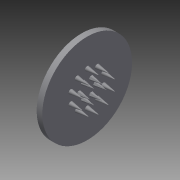
# Autodesk Inventor part: foam gripper
Saved by Autodesk Inventor 2015 (Build 190159000, 159)
## iProperties
Created: 2014-11-02
Part Number: foam gripper
Material: Generic
Document SubType Name: Modeling
Designer: jesse
Density: 1 g/cm^3
Appearance: Default
Author: jesse
Autodesk Inventor part; units mm, degrees
ref_plane "YZ Plane" through (0, 0, 0) normal (1, 0, 0) x (0, 1, 0)
ref_plane "XZ Plane" through (0, 0, 0) normal (0, 1, 0) x (-1, 0, 0)
ref_plane "XY Plane" through (0, 0, 0) normal (0, 0, 1) x (1, 0, 0)
sketch "Sketch1" plane through (0, 0, 0) normal (1, 0, 0) x (0, 1, 0)
  circle A0 centre (0, 0) radius 50.8
  dimension "d0" = 101.6
  constraints: 1 centre point, 1 coincident
  measures "d0" diameter of A0
extrude "Extrusion1" add sketch "Sketch1" along normal blind 3.175
sketch "Sketch2" plane through (3.175, 0, 0) normal (1, 0, 0) x (0, 0, -1)
  circle A0 centre (0, 19.4049) radius 2.54
  point P0 (0, 0)
  dimension "d3" = 5.08
  constraints: 1 centre point
  measures "d3" diameter of A0
extrude "Extrusion2" add sketch "Sketch2" along normal blind 12.7 draft -10
pattern_circular "Circular Pattern1" count 10 over 360 about axis through (0, 0, 0) along (1, 0, 0) of "Extrusion2"
sketch "Sketch3" plane through (3.175, 0, 0) normal (1, 0, 0) x (0, 0, -1)
  line L0 (6.7407, 0) -> (8.0059, 2.1913)
  line L1 (8.0059, 2.1913) -> (10.5361, 2.1913)
  line L2 (10.5361, 2.1913) -> (11.8012, 0)
  line L3 (11.8012, 0) -> (10.5361, -2.1913)
  line L4 (10.5361, -2.1913) -> (8.0059, -2.1913)
  line L5 (8.0059, -2.1913) -> (6.7407, 0)
  point P0 (0, 0)
  point P1 (9.271, 0)
  constraints: 12 end point, 13 other
extrude "Extrusion3" add sketch "Sketch3" along normal blind 12.7 draft -10
pattern_circular "Circular Pattern2" count 6 over 360 about axis through (0, 0, 0) along (1, 0, 0) of "Extrusion3"
sketch "Sketch4" plane through (3.175, 0, 0) normal (1, 0, 0) x (0, 0, -1)
  line L0 (-5.461, 3.1529) -> (0, 6.3058)
  line L1 (0, 6.3058) -> (5.461, 3.1529)
  line L2 (5.461, 3.1529) -> (5.461, -3.1529)
  line L3 (5.461, -3.1529) -> (0, -6.3058)
  line L4 (0, -6.3058) -> (-5.461, -3.1529)
  line L5 (-5.461, -3.1529) -> (-5.461, 3.1529)
  line L6 (-7.0782, -4.0866) -> (0, -8.1732)
  line L7 (0, -8.1732) -> (7.0782, -4.0866)
  line L8 (7.0782, -4.0866) -> (7.0782, 4.0866)
  line L9 (7.0782, 4.0866) -> (0, 8.1732)
  line L10 (0, 8.1732) -> (-7.0782, 4.0866)
  line L11 (-7.0782, 4.0866) -> (-7.0782, -4.0866)
  point P0 (0, 0)
  point P1 (0, 0)
  dimension "d14" = 10.922
  constraints: 24 end point, 1 coincident, 18 other
  measures "d14" distance between parallel lines of L1 L4
extrude "Extrusion4" add sketch "Sketch4" along normal blind 3.175
sketch "Sketch5" plane through (3.175, 0, 0) normal (1, 0, 0) x (0, 0, -1)
  circle A0 centre (0, 0) radius 3.175
  dimension "d17" = 6.35
  constraints: 1 centre point, 1 coincident
  measures "d17" diameter of A0
extrude "Extrusion5" cut sketch "Sketch5" against normal through all
body "Solid1"
